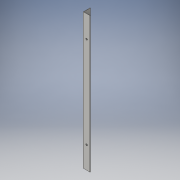
# Autodesk Inventor part: gripper main bracket
Saved by Autodesk Inventor 2016 SP2 (Build 200236200, 236)
## iProperties
Created: 2018-02-13
Part Number: gripper main bracket
Material: Generic
Document SubType Name: Modeling
Designer: CAD
Density: 1 g/cm^3
Appearance: Default
Author: CAD
Autodesk Inventor part; units mm, degrees
ref_plane "YZ Plane" through (0, 0, 0) normal (1, 0, 0) x (0, 1, 0)
ref_plane "XZ Plane" through (0, 0, 0) normal (0, 1, 0) x (-1, 0, 0)
ref_plane "XY Plane" through (0, 0, 0) normal (0, 0, 1) x (1, 0, 0)
sketch "Sketch1" plane through (0, 0, 0) normal (0, 1, 0) x (-1, 0, 0)
  line L0 (0, 0) -> (-25.4, 0)
  line L1 (0, 0) -> (0, -25.4)
  line L2 (-1.5875, -25.4) -> (-1.5875, -1.5875)
  line L3 (-1.5875, -1.5875) -> (-25.4, -1.5875)
  line L4 (0, -25.4) -> (-1.5875, -25.4)
  line L5 (-25.4, -1.5875) -> (-25.4, 0)
  dimension "d5" = 25.4
  dimension "d6" = 25.4
  dimension "d7" = 1.5875
  constraints: 12 end point, 2 perpendicular, 1 horizontal, 1 vertical, 1 other
  measures "d5" distance of L0.start L1.end
  measures "d6" distance of L0.start L0.end
  measures "d7" distance between parallel lines of L1 L2
extrude "Extrusion1" add sketch "Sketch1" along normal blind 508
sketch "Sketch2" plane through (25.4, 0, -1.5875) normal (0, 0, -1) x (-1, 0, 0)
  line L0 (0, 508) -> (23.8125, 508) projected
  line L1 (25.4, 0) -> (0, 0) projected
  line L2 (0, 0) -> (0, 508) projected
  point P0 (12.7, 425.45)
  point P1 (12.7, 82.55)
  dimension "d10" = 82.55
  dimension "d11" = 82.55
  dimension "d12" = 12.7
  dimension "d13" = 12.7
  measures "d10" distance from line of L0 point (12.7, 425.45)
  measures "d11" distance from line of L1 point (12.7, 82.55)
  measures "d12" distance from line of point (12.7, 82.55) L2
  measures "d13" distance from line of point (12.7, 425.45) L2
hole "Hole1" at (12.7, 425.45, -1.5875) at (12.7, 82.55, -1.5875) direction (0, 0, 1) diameter 6.35 end through all
body "Solid1"
